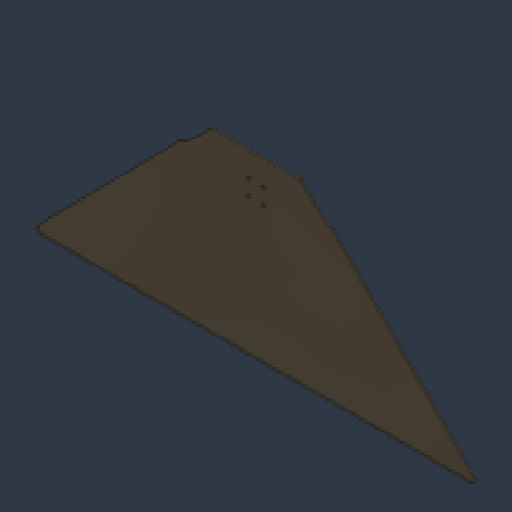
# Autodesk Inventor part: hopper_back_plate
Saved by Autodesk Inventor 2024.3 (Build 283343000, 343)
## iProperties
Created: 2025-03-05
Part Number: hopper_back_plate
Material: Polycarbonate, Smoke
Document SubType Name: Sheet Metal
Designer: Marcus Tannini
Density: 1.2 g/cm^3
Sheet Metal Rule: Default
Appearance: Polycarbonate - Smoked
Mass: 482.78 g
Surface Area: 2692.42 cm^2
Volume: 402.316 cm^3
Author: Marcus Tannini
Autodesk Inventor part; units mm, degrees
ref_plane "YZ Plane" through (0, 0, 0) normal (1, 0, 0) x (0, 1, 0)
ref_plane "XZ Plane" through (0, 0, 0) normal (0, 1, 0) x (-1, 0, 0)
ref_plane "XY Plane" through (0, 0, 0) normal (0, 0, 1) x (1, 0, 0)
sketch "Sketch1" plane through (0, 0, 0) normal (0, 0, 1) x (1, 0, 0)
  line L0 (381.5852, -185.7682) -> (94.217, 105.9508)
  line L1 (94.217, 105.9508) -> (-70.883, 105.9508)
  line L2 (-70.883, 105.9508) -> (-358.2512, -185.7682)
  line L3 (1105.6551, 353.06) -> (-810.8916, 353.06) construction
  line L4 (381.5852, -185.7682) -> (-358.2512, -185.7682)
  dimension "d4" = 165.1
  dimension "d7" = 291.719
  measures "d4" distance of L0.end L1.end
  measures "d7" distance between parallel lines of L4 L1
extrude "Plate1" add sketch "Sketch1" along normal blind 3.048
sketch "Sketch2" plane through (0, 0, 3.048) normal (0, 0, 1) x (1, 0, 0)
  line L0 (94.217, 105.9508) -> (381.5852, -185.7682) construction
  line L1 (-70.883, 105.9508) -> (94.217, 105.9508) construction
  line L2 (-358.2512, -185.7682) -> (-70.883, 105.9508) construction
  line L3 (381.5852, -185.7682) -> (-358.2512, -185.7682) construction
  line L4 (11.667, 105.9508) -> (11.667, -185.7682) construction
  point P0 (0, 0)
  point P1 (24.367, 64.6758)
  point P2 (24.367, 39.2758)
  point P3 (-1.033, 64.6758)
  point P4 (-1.033, 39.2758)
  dimension "d8" = 12.7
  dimension "d9" = 41.275
  dimension "d10" = 25.4
  constraints: 2 end point, 2 midpoint, 2 symmetric about line, 1 vertical alignment
  measures "d8" distance from line of L4 point (24.367, 64.676)
  measures "d9" distance from line of L1 point (24.367, 64.676)
  measures "d10" distance of point (24.367, 39.276) point (24.367, 64.676)
hole "Hole1" at (24.367, 64.6758, 3.048) at (24.367, 39.2758, 3.048) at (-1.033, 39.2758, 3.048) at (-1.033, 64.6758, 3.048) direction (0, 0, -1) diameter 5.1054 end through all clearance for "Flat Head Machine Screw (82)" size "#10" standard "Ansi Unified Screw Threads"
sketch "Sketch3" plane through (0, 0, 0) normal (0, 0, -1) x (-1, 0, 0)
  circle A0 centre (1.033, 64.6758) radius 2.5527 construction
  circle A1 centre (1.033, 39.2758) radius 2.5527 construction
  circle A2 centre (-24.367, 39.2758) radius 2.5527 construction
  circle A3 centre (-24.367, 64.6758) radius 2.5527 construction
  line L0 (-94.217, 105.9508) -> (70.883, 105.9508) projected
  line L1 (-381.5852, -185.7682) -> (-94.217, 105.9508) construction
  line L2 (358.2512, -185.7682) -> (-381.5852, -185.7682) construction
  line L3 (70.883, 105.9508) -> (358.2512, -185.7682) construction
  line L4 (115.4456, 60.7134) -> (110.9219, 56.2572)
  line L5 (110.9219, 56.2572) -> (66.3592, 101.4945)
  line L6 (66.3592, 101.4945) -> (70.883, 105.9508)
  line L7 (70.883, 105.9508) -> (115.4456, 60.7134)
  line L8 (66.3592, 101.4945) -> (61.9694, 105.9508)
  line L9 (-11.667, 105.9508) -> (-11.667, 80.5508) construction
  line L10 (-11.667, 105.9508) -> (13.733, 105.9508) construction
  line L11 (-138.7797, 60.7134) -> (-134.256, 56.2572)
  line L12 (-134.256, 56.2572) -> (-89.6933, 101.4945)
  line L13 (-94.217, 105.9508) -> (-138.7797, 60.7134)
  line L14 (-89.6933, 101.4945) -> (-85.3035, 105.9508)
  line L15 (-85.3035, 105.9508) -> (-134.256, 56.2572)
  line L16 (-134.256, 56.2572) -> (-138.7797, 60.7134)
  line L17 (-138.7797, 60.7134) -> (-94.217, 105.9508)
  line L18 (-94.217, 105.9508) -> (-85.3035, 105.9508)
  line L19 (70.883, 105.9508) -> (61.9694, 105.9508)
  point P0 (0, 0)
  dimension "d18" = 6.35
  dimension "d19" = 63.5
  dimension "d20" = 25.4
  dimension "d21" = 90
  constraints: 32 end point, 5 perpendicular, 4 collinear, 4 symmetric about line, 2 parallel, 2 point on line, 1 horizontal, 1 midpoint, 1 vertical
  measures "d18" distance of L4.start L4.end
  measures "d19" distance of L4.end L5.end
  measures "d20" distance of L9.start L9.end
  measures "d21" angle of L9 L10
extrude "Cut1" cut sketch "Sketch3" against normal blind 3.048
fillet "Corner Round1" radius 6.35 2 edges at (-358.2512, -185.7682, 1.524) (381.5852, -185.7682, 1.524)
fillet "Corner Round2" radius 127 2 edges at (-110.9219, 56.2572, 1.524) (134.256, 56.2572, 1.524)
equation "\"d16\" = Thickness"
equation "\"d22\" = Thickness"
equation "\"d2\" = Thickness"
equation "\"BendRadius\" = Thickness"
equation "\"BendReliefWidth\" = Thickness"
equation "\"BendReliefDepth\" = 0.5 * Thickness"
equation "\"CornerReliefSize\" = 4 * Thickness"
equation "\"MinimumRemnant\" = 2 * Thickness"
equation "\"TransitionRadius\" = BendRadius"
equation "\"JacobiRadiusSize\" = BendRadius"
equation "\"GapSize\" = Thickness"
equation "\"Thickness\" = 3.048"
body "Solid1"
